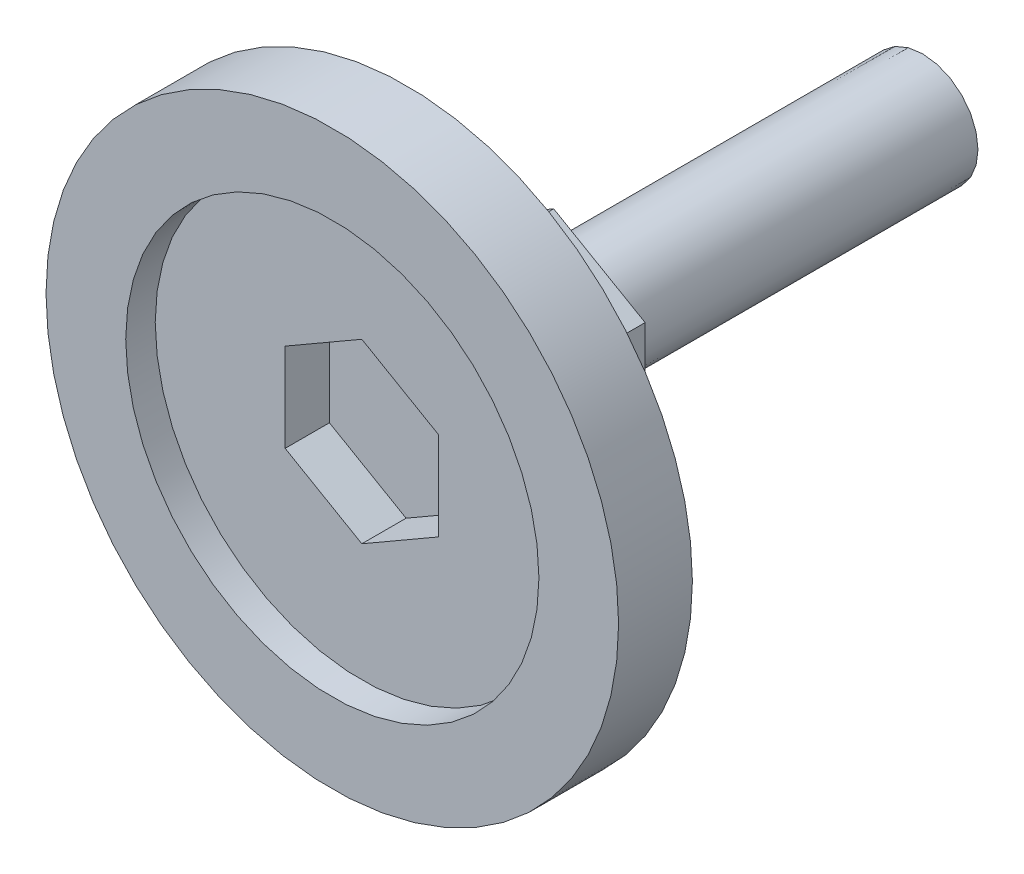
# Autodesk Inventor part: Reverser
Saved by Autodesk Inventor 2021 (Build 250183000, 183)
## iProperties
Created: 2021-07-06
Part Number: Reverser
Material: Generic
Document SubType Name: Modeling
Designer: teh18
Density: 1 g/cm^3
Appearance: Default
Author: teh18
Autodesk Inventor part; units mm, degrees
sketch "Sketch1" plane through (0, 0, 0) normal (0, 0, 1) x (1, 0, 0)
  circle A0 centre (0, 0) radius 19.4
  circle A1 centre (0, 0) radius 14
  dimension "d0" = 38.8
  dimension "d1" = 28
  constraints: 2 centre point, 2 coincident
  measures "d0" diameter of A0
  measures "d1" diameter of A1
extrude "Extrusion1" add sketch "Sketch1" against normal blind 2
ref_plane "Work Plane1" through (-19.6075, -25, -15) normal (0, 0, 1) x (1, 0, 0)
ref_plane "Work Plane2" through (-137.3725, -100, -40) normal (0, 0, -1) x (0, 1, 0)
sketch "Sketch5" plane through (0, 0, -2) normal (0, 0, -1) x (-1, 0, 0)
  circle A0 centre (0, 0) radius 19.4 projected
  line L0 (-5.1962, -3) -> (-5.1962, 3)
  line L1 (-5.1962, 3) -> (0, 6)
  line L2 (0, 6) -> (5.1962, 3)
  line L3 (5.1962, 3) -> (5.1962, -3)
  line L4 (5.1962, -3) -> (0, -6)
  line L5 (0, -6) -> (-5.1962, -3)
  dimension "d14" = 6
  constraints: 12 end point, 1 coincident, 1 vertical alignment, 13 other
  measures "d14" distance of L0.start L0.end
extrude "Extrusion5" add sketch "Sketch5" along normal blind 3
sketch "Sketch6" plane through (0, 0, -5) normal (0, 0, -1) x (-1, 0, 0)
  circle A0 centre (0, 0) radius 19.4 projected
  line L0 (-5.1962, -3) -> (-5.1962, 3) projected
  line L1 (-5.1962, 3) -> (0, 6) projected
  line L2 (0, 6) -> (5.1962, 3) projected
  line L3 (5.1962, 3) -> (5.1962, -3) projected
  line L4 (5.1962, -3) -> (0, -6) projected
  line L5 (0, -6) -> (-5.1962, -3) projected
  line L6 (-6.1962, 3.5774) -> (-6.1962, -3.5774)
  line L7 (-6.1962, -3.5774) -> (0, -7.1547)
  line L8 (0, -7.1547) -> (6.1962, -3.5774)
  line L9 (6.1962, -3.5774) -> (6.1962, 3.5774)
  line L10 (6.1962, 3.5774) -> (0, 7.1547)
  line L11 (0, 7.1547) -> (-6.1962, 3.5774)
  dimension "d17" = 1
  constraints: 12 end point, 5 other
  measures "d17" distance between parallel lines of L0 L6
ref_plane "Work Plane3" through (-19.6075, -25, -15) normal (0, 0, 1) x (1, 0, 0)
extrude "Extrusion6" add sketch "Sketch6" along normal up to surface (10 mm away) contours L0 L1 L2 L3 L4 L5 | L11 L10 L9 L8 L7 L6
sketch "Sketch7" plane through (6.1962, -3.5774, -15) normal (0, 0, -1) x (-1, 0, 0)
  circle A0 centre (6.1962, 3.5774) radius 3.75
  dimension "d20" = 7.5
  constraints: 1 centre point, 1 coincident
  measures "d20" diameter of A0
ref_plane "Work Plane4" through (-137.3725, -100, -40) normal (0, 0, -1) x (0, 1, 0)
extrude "Extrusion7" add sketch "Sketch7" along normal up to surface (25 mm away)
body "Solid1"
